Autodesk Inventor part; units mm, degrees
(part 2 of 2)
sketch "Sketch4" plane through (0, 0, 20) normal (0, 0, 1) x (1, 0, 0)
  line L0 (-68.9429, 68.9429) -> (-21.2132, 21.2132) projected
  arc A0 (-21.2132, 21.2132) -> (21.2132, -21.2132) centre (0, 0) ccw projected
  line L1 (21.2132, -21.2132) -> (68.9429, -68.9429) projected
  arc A1 (68.9429, -68.9429) -> (69.4823, -68.3993) centre (0, 0) ccw projected
  arc A2 (69.4823, -68.3993) -> (73.8041, -70.4056) centre (83.4681, -43.9299) ccw projected
  arc A3 (73.8041, -70.4056) -> (74.9009, -69.2377) centre (0, 0) ccw projected
  arc A4 (74.9009, -69.2377) -> (72.6272, -65.0503) centre (49.0843, -80.5451) ccw projected
  arc A5 (72.6272, -65.0503) -> (73.64, -63.9015) centre (0, 0) ccw projected
  arc A6 (73.64, -63.9015) -> (78.0793, -65.6325) centre (86.0618, -38.6023) ccw projected
  arc A7 (78.0793, -65.6325) -> (79.1006, -64.398) centre (0, 0) ccw projected
  arc A8 (79.1006, -64.398) -> (76.5684, -60.3617) centre (54.0449, -77.3041) ccw projected
  arc A9 (76.5684, -60.3617) -> (77.5071, -59.1515) centre (0, 0) ccw projected
  arc A10 (77.5071, -59.1515) -> (82.0463, -60.6003) centre (88.3159, -33.1222) ccw projected
  arc A11 (82.0463, -60.6003) -> (82.9881, -59.3041) centre (0, 0) ccw projected
  arc A12 (82.9881, -59.3041) -> (80.2075, -55.4348) centre (58.7922, -73.758) ccw projected
  arc A13 (80.2075, -55.4348) -> (81.0683, -54.1681) centre (0, 0) ccw projected
  arc A14 (81.0683, -54.1681) -> (85.6895, -55.329) centre (90.2213, -27.5115) ccw projected
  arc A15 (85.6895, -55.329) -> (86.548, -53.9763) centre (0, 0) ccw projected
  arc A16 (86.548, -53.9763) -> (83.53, -50.2891) centre (63.3075, -69.9209) ccw projected
  arc A17 (83.53, -50.2891) -> (84.3096, -48.9709) centre (0, 0) ccw projected
  arc A18 (84.3096, -48.9709) -> (88.9946, -49.8394) centre (91.7708, -21.7921) ccw projected
  arc A19 (88.9946, -49.8394) -> (89.7665, -48.4354) centre (0, 0) ccw projected
  arc A20 (89.7665, -48.4354) -> (86.5228, -44.945) centre (67.5729, -65.8078) ccw projected
  arc A21 (86.5228, -44.945) -> (87.2181, -43.5804) centre (0, 0) ccw projected
  arc A22 (87.2181, -43.5804) -> (91.9484, -44.153) centre (92.958, -15.9868) ccw projected
  arc A23 (91.9484, -44.153) -> (92.6306, -42.7033) centre (0, 0) ccw projected
  arc A24 (92.6306, -42.7033) -> (89.1742, -39.4235) centre (71.5717, -61.435) ccw projected
  arc A25 (89.1742, -39.4235) -> (89.7824, -38.0179) centre (0, 0) ccw projected
  arc A26 (89.7824, -38.0179) -> (94.5394, -38.2924) centre (93.7784, -10.1184) ccw projected
  arc A27 (94.5394, -38.2924) -> (95.1292, -36.8027) centre (0, 0) ccw projected
  arc A28 (95.1292, -36.8027) -> (91.4737, -33.7464) centre (75.288, -56.8198) ccw projected
  arc A29 (91.4737, -33.7464) -> (91.9924, -32.3054) centre (0, 0) ccw projected
  arc A30 (91.9924, -32.3054) -> (96.7572, -32.2807) centre (94.2287, -4.21) ccw projected
  arc A31 (96.7572, -32.2807) -> (97.2523, -30.7569) centre (0, 0) ccw projected
  arc A32 (97.2523, -30.7569) -> (93.4121, -27.9361) centre (78.7072, -51.9803) ccw projected
  arc A33 (93.4121, -27.9361) -> (93.8394, -26.4654) centre (0, 0) ccw projected
  arc A34 (93.8394, -26.4654) -> (98.5932, -26.1415) centre (94.3071, 1.715) ccw projected
  arc A35 (98.5932, -26.1415) -> (98.9917, -24.5897) centre (0, 0) ccw projected
  arc A36 (98.9917, -24.5897) -> (94.9819, -22.0156) centre (81.8157, -46.9356) ccw projected
  arc A37 (94.9819, -22.0156) -> (95.316, -20.521) centre (0, 0) ccw projected
  arc A38 (95.316, -20.521) -> (100.0401, -19.8992) centre (94.0133, 7.6332) ccw projected
  arc A39 (100.0401, -19.8992) -> (100.3403, -18.3254) centre (0, 0) ccw projected
  arc A40 (100.3403, -18.3254) -> (96.1769, -16.0082) centre (84.6014, -41.7058) ccw projected
  arc A41 (96.1769, -16.0082) -> (96.4164, -14.4956) centre (0, 0) ccw projected
  arc A42 (96.4164, -14.4956) -> (101.0922, -13.5784) centre (93.3485, 13.5213) ccw projected
  arc A43 (101.0922, -13.5784) -> (101.293, -11.9888) centre (0, 0) ccw projected
  arc A44 (101.293, -11.9888) -> (96.9922, -9.9376) centre (87.0532, -36.3113) ccw projected
  arc A45 (96.9922, -9.9376) -> (97.1364, -8.4129) centre (0, 0) ccw projected
  arc A46 (97.1364, -8.4129) -> (101.7453, -7.204) centre (92.3153, 19.356) ccw projected
  arc A47 (101.7453, -7.204) -> (101.8459, -5.6049) centre (0, 0) ccw projected
  arc A48 (101.8459, -5.6049) -> (97.4248, -3.8278) centre (89.1614, -30.7735) ccw projected
  arc A49 (97.4248, -3.8278) -> (97.4729, -2.2971) centre (0, 0) ccw projected
  arc A50 (97.4729, -2.2971) -> (101.9969, -0.8011) centre (90.9178, 25.1143) ccw projected
  arc A51 (101.9969, -0.8011) -> (101.9969, 0.8011) centre (0, 0) ccw projected
  arc A52 (101.9969, 0.8011) -> (97.4729, 2.2971) centre (90.9178, -25.1143) ccw projected
  arc A53 (97.4729, 2.2971) -> (97.4248, 3.8278) centre (0, 0) ccw projected
  arc A54 (97.4248, 3.8278) -> (101.8459, 5.6049) centre (89.1614, 30.7735) ccw projected
  arc A55 (101.8459, 5.6049) -> (101.7453, 7.204) centre (0, 0) ccw projected
  arc A56 (101.7453, 7.204) -> (97.1364, 8.4129) centre (92.3153, -19.356) ccw projected
  arc A57 (97.1364, 8.4129) -> (96.9922, 9.9376) centre (0, 0) ccw projected
  arc A58 (96.9922, 9.9376) -> (101.293, 11.9888) centre (87.0532, 36.3113) ccw projected
  arc A59 (101.293, 11.9888) -> (101.0922, 13.5784) centre (0, 0) ccw projected
  arc A60 (101.0922, 13.5784) -> (96.4164, 14.4956) centre (93.3485, -13.5213) ccw projected
  arc A61 (96.4164, 14.4956) -> (96.1769, 16.0082) centre (0, 0) ccw projected
  arc A62 (96.1769, 16.0082) -> (100.3403, 18.3254) centre (84.6014, 41.7058) ccw projected
  arc A63 (100.3403, 18.3254) -> (100.0401, 19.8992) centre (0, 0) ccw projected
  arc A64 (100.0401, 19.8992) -> (95.316, 20.521) centre (94.0133, -7.6332) ccw projected
  arc A65 (95.316, 20.521) -> (94.9819, 22.0156) centre (0, 0) ccw projected
  arc A66 (94.9819, 22.0156) -> (98.9917, 24.5897) centre (81.8157, 46.9356) ccw projected
  arc A67 (98.9917, 24.5897) -> (98.5932, 26.1415) centre (0, 0) ccw projected
  arc A68 (98.5932, 26.1415) -> (93.8394, 26.4654) centre (94.3071, -1.715) ccw projected
  arc A69 (93.8394, 26.4654) -> (93.4121, 27.9361) centre (0, 0) ccw projected
  arc A70 (93.4121, 27.9361) -> (97.2523, 30.7569) centre (78.7072, 51.9803) ccw projected
  arc A71 (97.2523, 30.7569) -> (96.7572, 32.2807) centre (0, 0) ccw projected
  arc A72 (96.7572, 32.2807) -> (91.9924, 32.3054) centre (94.2287, 4.21) ccw projected
  arc A73 (91.9924, 32.3054) -> (91.4737, 33.7464) centre (0, 0) ccw projected
  arc A74 (91.4737, 33.7464) -> (95.1292, 36.8027) centre (75.288, 56.8198) ccw projected
  arc A75 (95.1292, 36.8027) -> (94.5394, 38.2924) centre (0, 0) ccw projected
  arc A76 (94.5394, 38.2924) -> (89.7824, 38.0179) centre (93.7784, 10.1184) ccw projected
  arc A77 (89.7824, 38.0179) -> (89.1742, 39.4235) centre (0, 0) ccw projected
  arc A78 (89.1742, 39.4235) -> (92.6306, 42.7033) centre (71.5717, 61.435) ccw projected
  arc A79 (92.6306, 42.7033) -> (91.9484, 44.153) centre (0, 0) ccw projected
  arc A80 (91.9484, 44.153) -> (87.2181, 43.5804) centre (92.958, 15.9868) ccw projected
  arc A81 (87.2181, 43.5804) -> (86.5228, 44.945) centre (0, 0) ccw projected
  arc A82 (86.5228, 44.945) -> (89.7665, 48.4354) centre (67.5729, 65.8078) ccw projected
  arc A83 (89.7665, 48.4354) -> (88.9946, 49.8394) centre (0, 0) ccw projected
  arc A84 (88.9946, 49.8394) -> (84.3096, 48.9709) centre (91.7708, 21.7921) ccw projected
  arc A85 (84.3096, 48.9709) -> (83.53, 50.2891) centre (0, 0) ccw projected
  arc A86 (83.53, 50.2891) -> (86.548, 53.9763) centre (63.3075, 69.9209) ccw projected
  arc A87 (86.548, 53.9763) -> (85.6895, 55.329) centre (0, 0) ccw projected
  arc A88 (85.6895, 55.329) -> (81.0683, 54.1681) centre (90.2213, 27.5115) ccw projected
  arc A89 (81.0683, 54.1681) -> (80.2075, 55.4348) centre (0, 0) ccw projected
  arc A90 (80.2075, 55.4348) -> (82.9881, 59.3041) centre (58.7922, 73.758) ccw projected
  arc A91 (82.9881, 59.3041) -> (82.0463, 60.6003) centre (0, 0) ccw projected
  arc A92 (82.0463, 60.6003) -> (77.5071, 59.1515) centre (88.3159, 33.1222) ccw projected
  arc A93 (77.5071, 59.1515) -> (76.5684, 60.3617) centre (0, 0) ccw projected
  arc A94 (76.5684, 60.3617) -> (79.1006, 64.398) centre (54.0449, 77.3041) ccw projected
  arc A95 (79.1006, 64.398) -> (78.0793, 65.6325) centre (0, 0) ccw projected
  arc A96 (78.0793, 65.6325) -> (73.64, 63.9015) centre (86.0618, 38.6023) ccw projected
  arc A97 (73.64, 63.9015) -> (72.6272, 65.0503) centre (0, 0) ccw projected
  arc A98 (72.6272, 65.0503) -> (74.9009, 69.2377) centre (49.0843, 80.5451) ccw projected
  arc A99 (74.9009, 69.2377) -> (73.8041, 70.4056) centre (0, 0) ccw projected
  arc A100 (73.8041, 70.4056) -> (69.4823, 68.3993) centre (83.4681, 43.9299) ccw projected
  arc A101 (69.4823, 68.3993) -> (68.3993, 69.4823) centre (0, 0) ccw projected
  arc A102 (68.3993, 69.4823) -> (70.4056, 73.8041) centre (43.9299, 83.4681) ccw projected
  arc A103 (70.4056, 73.8041) -> (69.2377, 74.9009) centre (0, 0) ccw projected
  arc A104 (69.2377, 74.9009) -> (65.0503, 72.6272) centre (80.5451, 49.0843) ccw projected
  arc A105 (65.0503, 72.6272) -> (63.9015, 73.64) centre (0, 0) ccw projected
  arc A106 (63.9015, 73.64) -> (65.6325, 78.0793) centre (38.6023, 86.0618) ccw projected
  arc A107 (65.6325, 78.0793) -> (64.398, 79.1006) centre (0, 0) ccw projected
  arc A108 (64.398, 79.1006) -> (60.3617, 76.5684) centre (77.3041, 54.0449) ccw projected
  arc A109 (60.3617, 76.5684) -> (59.1515, 77.5071) centre (0, 0) ccw projected
  arc A110 (59.1515, 77.5071) -> (60.6003, 82.0463) centre (33.1222, 88.3159) ccw projected
  arc A111 (60.6003, 82.0463) -> (59.3041, 82.9881) centre (0, 0) ccw projected
  arc A112 (59.3041, 82.9881) -> (55.4348, 80.2075) centre (73.758, 58.7922) ccw projected
  arc A113 (55.4348, 80.2075) -> (54.1681, 81.0683) centre (0, 0) ccw projected
  arc A114 (54.1681, 81.0683) -> (55.329, 85.6895) centre (27.5115, 90.2213) ccw projected
  arc A115 (55.329, 85.6895) -> (53.9763, 86.548) centre (0, 0) ccw projected
  arc A116 (53.9763, 86.548) -> (50.2891, 83.53) centre (69.9209, 63.3075) ccw projected
  arc A117 (50.2891, 83.53) -> (48.9709, 84.3096) centre (0, 0) ccw projected
  arc A118 (48.9709, 84.3096) -> (49.8394, 88.9946) centre (21.7921, 91.7708) ccw projected
  arc A119 (49.8394, 88.9946) -> (48.4354, 89.7665) centre (0, 0) ccw projected
  arc A120 (48.4354, 89.7665) -> (44.945, 86.5228) centre (65.8078, 67.5729) ccw projected
  arc A121 (44.945, 86.5228) -> (43.5804, 87.2181) centre (0, 0) ccw projected
  arc A122 (43.5804, 87.2181) -> (44.153, 91.9484) centre (15.9868, 92.958) ccw projected
  arc A123 (44.153, 91.9484) -> (42.7033, 92.6306) centre (0, 0) ccw projected
  arc A124 (42.7033, 92.6306) -> (39.4235, 89.1742) centre (61.435, 71.5717) ccw projected
  arc A125 (39.4235, 89.1742) -> (38.0179, 89.7824) centre (0, 0) ccw projected
  arc A126 (38.0179, 89.7824) -> (38.2924, 94.5394) centre (10.1184, 93.7784) ccw projected
  arc A127 (38.2924, 94.5394) -> (36.8027, 95.1292) centre (0, 0) ccw projected
  arc A128 (36.8027, 95.1292) -> (33.7464, 91.4737) centre (56.8198, 75.288) ccw projected
  arc A129 (33.7464, 91.4737) -> (32.3054, 91.9924) centre (0, 0) ccw projected
  arc A130 (32.3054, 91.9924) -> (32.2807, 96.7572) centre (4.21, 94.2287) ccw projected
  arc A131 (32.2807, 96.7572) -> (30.7569, 97.2523) centre (0, 0) ccw projected
  arc A132 (30.7569, 97.2523) -> (27.9361, 93.4121) centre (51.9803, 78.7072) ccw projected
  arc A133 (27.9361, 93.4121) -> (26.4654, 93.8394) centre (0, 0) ccw projected
  arc A134 (26.4654, 93.8394) -> (26.1415, 98.5932) centre (-1.715, 94.3071) ccw projected
  arc A135 (26.1415, 98.5932) -> (24.5897, 98.9917) centre (0, 0) ccw projected
  arc A136 (24.5897, 98.9917) -> (22.0156, 94.9819) centre (46.9356, 81.8157) ccw projected
  arc A137 (22.0156, 94.9819) -> (20.521, 95.316) centre (0, 0) ccw projected
  arc A138 (20.521, 95.316) -> (19.8992, 100.0401) centre (-7.6332, 94.0133) ccw projected
  arc A139 (19.8992, 100.0401) -> (18.3254, 100.3403) centre (0, 0) ccw projected
  arc A140 (18.3254, 100.3403) -> (16.0082, 96.1769) centre (41.7058, 84.6014) ccw projected
  arc A141 (16.0082, 96.1769) -> (14.4956, 96.4164) centre (0, 0) ccw projected
  arc A142 (14.4956, 96.4164) -> (13.5784, 101.0922) centre (-13.5213, 93.3485) ccw projected
  arc A143 (13.5784, 101.0922) -> (11.9888, 101.293) centre (0, 0) ccw projected
  arc A144 (11.9888, 101.293) -> (9.9376, 96.9922) centre (36.3113, 87.0532) ccw projected
  arc A145 (9.9376, 96.9922) -> (8.4129, 97.1364) centre (0, 0) ccw projected
  arc A146 (8.4129, 97.1364) -> (7.204, 101.7453) centre (-19.356, 92.3153) ccw projected
  arc A147 (7.204, 101.7453) -> (5.6049, 101.8459) centre (0, 0) ccw projected
  arc A148 (5.6049, 101.8459) -> (3.8278, 97.4248) centre (30.7735, 89.1614) ccw projected
  arc A149 (3.8278, 97.4248) -> (2.2971, 97.4729) centre (0, 0) ccw projected
  arc A150 (2.2971, 97.4729) -> (0.8011, 101.9969) centre (-25.1143, 90.9178) ccw projected
  arc A151 (0.8011, 101.9969) -> (-0.8011, 101.9969) centre (0, 0) ccw projected
  arc A152 (-0.8011, 101.9969) -> (-2.2971, 97.4729) centre (25.1143, 90.9178) ccw projected
  arc A153 (-2.2971, 97.4729) -> (-3.8278, 97.4248) centre (0, 0) ccw projected
  arc A154 (-3.8278, 97.4248) -> (-5.6049, 101.8459) centre (-30.7735, 89.1614) ccw projected
  arc A155 (-5.6049, 101.8459) -> (-7.204, 101.7453) centre (0, 0) ccw projected
  arc A156 (-7.204, 101.7453) -> (-8.4129, 97.1364) centre (19.356, 92.3153) ccw projected
  arc A157 (-8.4129, 97.1364) -> (-9.9376, 96.9922) centre (0, 0) ccw projected
  arc A158 (-9.9376, 96.9922) -> (-11.9888, 101.293) centre (-36.3113, 87.0532) ccw projected
  arc A159 (-11.9888, 101.293) -> (-13.5784, 101.0922) centre (0, 0) ccw projected
  arc A160 (-13.5784, 101.0922) -> (-14.4956, 96.4164) centre (13.5213, 93.3485) ccw projected
  arc A161 (-14.4956, 96.4164) -> (-16.0082, 96.1769) centre (0, 0) ccw projected
  arc A162 (-16.0082, 96.1769) -> (-18.3254, 100.3403) centre (-41.7058, 84.6014) ccw projected
  arc A163 (-18.3254, 100.3403) -> (-19.8992, 100.0401) centre (0, 0) ccw projected
  arc A164 (-19.8992, 100.0401) -> (-20.521, 95.316) centre (7.6332, 94.0133) ccw projected
  arc A165 (-20.521, 95.316) -> (-22.0156, 94.9819) centre (0, 0) ccw projected
  arc A166 (-22.0156, 94.9819) -> (-24.5897, 98.9917) centre (-46.9356, 81.8157) ccw projected
  arc A167 (-24.5897, 98.9917) -> (-26.1415, 98.5932) centre (0, 0) ccw projected
  arc A168 (-26.1415, 98.5932) -> (-26.4654, 93.8394) centre (1.715, 94.3071) ccw projected
  arc A169 (-26.4654, 93.8394) -> (-27.9361, 93.4121) centre (0, 0) ccw projected
  arc A170 (-27.9361, 93.4121) -> (-30.7569, 97.2523) centre (-51.9803, 78.7072) ccw projected
  arc A171 (-30.7569, 97.2523) -> (-32.2807, 96.7572) centre (0, 0) ccw projected
  arc A172 (-32.2807, 96.7572) -> (-32.3054, 91.9924) centre (-4.21, 94.2287) ccw projected
  arc A173 (-32.3054, 91.9924) -> (-33.7464, 91.4737) centre (0, 0) ccw projected
  arc A174 (-33.7464, 91.4737) -> (-36.8027, 95.1292) centre (-56.8198, 75.288) ccw projected
  arc A175 (-36.8027, 95.1292) -> (-38.2924, 94.5394) centre (0, 0) ccw projected
  arc A176 (-38.2924, 94.5394) -> (-38.0179, 89.7824) centre (-10.1184, 93.7784) ccw projected
  arc A177 (-38.0179, 89.7824) -> (-39.4235, 89.1742) centre (0, 0) ccw projected
  arc A178 (-39.4235, 89.1742) -> (-42.7033, 92.6306) centre (-61.435, 71.5717) ccw projected
  arc A179 (-42.7033, 92.6306) -> (-44.153, 91.9484) centre (0, 0) ccw projected
  arc A180 (-44.153, 91.9484) -> (-43.5804, 87.2181) centre (-15.9868, 92.958) ccw projected
  arc A181 (-43.5804, 87.2181) -> (-44.945, 86.5228) centre (0, 0) ccw projected
  arc A182 (-44.945, 86.5228) -> (-48.4354, 89.7665) centre (-65.8078, 67.5729) ccw projected
  arc A183 (-48.4354, 89.7665) -> (-49.8394, 88.9946) centre (0, 0) ccw projected
  arc A184 (-49.8394, 88.9946) -> (-48.9709, 84.3096) centre (-21.7921, 91.7708) ccw projected
  arc A185 (-48.9709, 84.3096) -> (-50.2891, 83.53) centre (0, 0) ccw projected
  arc A186 (-50.2891, 83.53) -> (-53.9763, 86.548) centre (-69.9209, 63.3075) ccw projected
  arc A187 (-53.9763, 86.548) -> (-55.329, 85.6895) centre (0, 0) ccw projected
  arc A188 (-55.329, 85.6895) -> (-54.1681, 81.0683) centre (-27.5115, 90.2213) ccw projected
  arc A189 (-54.1681, 81.0683) -> (-55.4348, 80.2075) centre (0, 0) ccw projected
  arc A190 (-55.4348, 80.2075) -> (-59.3041, 82.9881) centre (-73.758, 58.7922) ccw projected
  arc A191 (-59.3041, 82.9881) -> (-60.6003, 82.0463) centre (0, 0) ccw projected
  arc A192 (-60.6003, 82.0463) -> (-59.1515, 77.5071) centre (-33.1222, 88.3159) ccw projected
  arc A193 (-59.1515, 77.5071) -> (-60.3617, 76.5684) centre (0, 0) ccw projected
  arc A194 (-60.3617, 76.5684) -> (-64.398, 79.1006) centre (-77.3041, 54.0449) ccw projected
  arc A195 (-64.398, 79.1006) -> (-65.6325, 78.0793) centre (0, 0) ccw projected
  arc A196 (-65.6325, 78.0793) -> (-63.9015, 73.64) centre (-38.6023, 86.0618) ccw projected
  arc A197 (-63.9015, 73.64) -> (-65.0503, 72.6272) centre (0, 0) ccw projected
  arc A198 (-65.0503, 72.6272) -> (-69.2377, 74.9009) centre (-80.5451, 49.0843) ccw projected
  arc A199 (-69.2377, 74.9009) -> (-70.4056, 73.8041) centre (0, 0) ccw projected
  arc A200 (-70.4056, 73.8041) -> (-68.3993, 69.4823) centre (-43.9299, 83.4681) ccw projected
  arc A201 (-68.3993, 69.4823) -> (-68.9429, 68.9429) centre (0, 0) ccw projected
  circle A202 centre (0, 0) radius 10 projected
  line L2 (0, 0) -> (21.2132, 21.2132)
  line L3 (0, 0) -> (30, 0) construction
  circle A203 centre (21.2132, 21.2132) radius 10
  dimension "d55" = 30
  dimension "d56" = 45
  dimension "d57" = 20
  constraints: 4 end point, 1 centre point, 1 coincident, 1 equal length, 1 horizontal
  measures "d55" distance of L2.start L2.end
  measures "d56" angle of L3 L2
  measures "d57" diameter of A203
extrude "Extrusion3" cut sketch "Sketch4" against normal up to surface (20 mm away) contours A203
sketch "Sketch6" plane through (0, 0, 20) normal (0, 0, 1) x (1, 0, 0)
  circle A0 centre (21.2132, 21.2132) radius 10 projected
  line L0 (-68.9429, 68.9429) -> (-21.2132, 21.2132) projected
  arc A1 (-21.2132, 21.2132) -> (21.2132, -21.2132) centre (0, 0) ccw projected
  line L1 (21.2132, -21.2132) -> (68.9429, -68.9429) projected
  arc A2 (68.9429, -68.9429) -> (69.4823, -68.3993) centre (0, 0) ccw projected
  arc A3 (69.4823, -68.3993) -> (73.8041, -70.4056) centre (83.4681, -43.9299) ccw projected
  arc A4 (73.8041, -70.4056) -> (74.9009, -69.2377) centre (0, 0) ccw projected
  arc A5 (74.9009, -69.2377) -> (72.6272, -65.0503) centre (49.0843, -80.5451) ccw projected
  arc A6 (72.6272, -65.0503) -> (73.64, -63.9015) centre (0, 0) ccw projected
  arc A7 (73.64, -63.9015) -> (78.0793, -65.6325) centre (86.0618, -38.6023) ccw projected
  arc A8 (78.0793, -65.6325) -> (79.1006, -64.398) centre (0, 0) ccw projected
  arc A9 (79.1006, -64.398) -> (76.5684, -60.3617) centre (54.0449, -77.3041) ccw projected
  arc A10 (76.5684, -60.3617) -> (77.5071, -59.1515) centre (0, 0) ccw projected
  arc A11 (77.5071, -59.1515) -> (82.0463, -60.6003) centre (88.3159, -33.1222) ccw projected
  arc A12 (82.0463, -60.6003) -> (82.9881, -59.3041) centre (0, 0) ccw projected
  arc A13 (82.9881, -59.3041) -> (80.2075, -55.4348) centre (58.7922, -73.758) ccw projected
  arc A14 (80.2075, -55.4348) -> (81.0683, -54.1681) centre (0, 0) ccw projected
  arc A15 (81.0683, -54.1681) -> (85.6895, -55.329) centre (90.2213, -27.5115) ccw projected
  arc A16 (85.6895, -55.329) -> (86.548, -53.9763) centre (0, 0) ccw projected
  arc A17 (86.548, -53.9763) -> (83.53, -50.2891) centre (63.3075, -69.9209) ccw projected
  arc A18 (83.53, -50.2891) -> (84.3096, -48.9709) centre (0, 0) ccw projected
  arc A19 (84.3096, -48.9709) -> (88.9946, -49.8394) centre (91.7708, -21.7921) ccw projected
  arc A20 (88.9946, -49.8394) -> (89.7665, -48.4354) centre (0, 0) ccw projected
  arc A21 (89.7665, -48.4354) -> (86.5228, -44.945) centre (67.5729, -65.8078) ccw projected
  arc A22 (86.5228, -44.945) -> (87.2181, -43.5804) centre (0, 0) ccw projected
  arc A23 (87.2181, -43.5804) -> (91.9484, -44.153) centre (92.958, -15.9868) ccw projected
  arc A24 (91.9484, -44.153) -> (92.6306, -42.7033) centre (0, 0) ccw projected
  arc A25 (92.6306, -42.7033) -> (89.1742, -39.4235) centre (71.5717, -61.435) ccw projected
  arc A26 (89.1742, -39.4235) -> (89.7824, -38.0179) centre (0, 0) ccw projected
  arc A27 (89.7824, -38.0179) -> (94.5394, -38.2924) centre (93.7784, -10.1184) ccw projected
  arc A28 (94.5394, -38.2924) -> (95.1292, -36.8027) centre (0, 0) ccw projected
  arc A29 (95.1292, -36.8027) -> (91.4737, -33.7464) centre (75.288, -56.8198) ccw projected
  arc A30 (91.4737, -33.7464) -> (91.9924, -32.3054) centre (0, 0) ccw projected
  arc A31 (91.9924, -32.3054) -> (96.7572, -32.2807) centre (94.2287, -4.21) ccw projected
  arc A32 (96.7572, -32.2807) -> (97.2523, -30.7569) centre (0, 0) ccw projected
  arc A33 (97.2523, -30.7569) -> (93.4121, -27.9361) centre (78.7072, -51.9803) ccw projected
  arc A34 (93.4121, -27.9361) -> (93.8394, -26.4654) centre (0, 0) ccw projected
  arc A35 (93.8394, -26.4654) -> (98.5932, -26.1415) centre (94.3071, 1.715) ccw projected
  arc A36 (98.5932, -26.1415) -> (98.9917, -24.5897) centre (0, 0) ccw projected
  arc A37 (98.9917, -24.5897) -> (94.9819, -22.0156) centre (81.8157, -46.9356) ccw projected
  arc A38 (94.9819, -22.0156) -> (95.316, -20.521) centre (0, 0) ccw projected
  arc A39 (95.316, -20.521) -> (100.0401, -19.8992) centre (94.0133, 7.6332) ccw projected
  arc A40 (100.0401, -19.8992) -> (100.3403, -18.3254) centre (0, 0) ccw projected
  arc A41 (100.3403, -18.3254) -> (96.1769, -16.0082) centre (84.6014, -41.7058) ccw projected
  arc A42 (96.1769, -16.0082) -> (96.4164, -14.4956) centre (0, 0) ccw projected
  arc A43 (96.4164, -14.4956) -> (101.0922, -13.5784) centre (93.3485, 13.5213) ccw projected
  arc A44 (101.0922, -13.5784) -> (101.293, -11.9888) centre (0, 0) ccw projected
  arc A45 (101.293, -11.9888) -> (96.9922, -9.9376) centre (87.0532, -36.3113) ccw projected
  arc A46 (96.9922, -9.9376) -> (97.1364, -8.4129) centre (0, 0) ccw projected
  arc A47 (97.1364, -8.4129) -> (101.7453, -7.204) centre (92.3153, 19.356) ccw projected
  arc A48 (101.7453, -7.204) -> (101.8459, -5.6049) centre (0, 0) ccw projected
  arc A49 (101.8459, -5.6049) -> (97.4248, -3.8278) centre (89.1614, -30.7735) ccw projected
  arc A50 (97.4248, -3.8278) -> (97.4729, -2.2971) centre (0, 0) ccw projected
  arc A51 (97.4729, -2.2971) -> (101.9969, -0.8011) centre (90.9178, 25.1143) ccw projected
  arc A52 (101.9969, -0.8011) -> (101.9969, 0.8011) centre (0, 0) ccw projected
  arc A53 (101.9969, 0.8011) -> (97.4729, 2.2971) centre (90.9178, -25.1143) ccw projected
  arc A54 (97.4729, 2.2971) -> (97.4248, 3.8278) centre (0, 0) ccw projected
  arc A55 (97.4248, 3.8278) -> (101.8459, 5.6049) centre (89.1614, 30.7735) ccw projected
  arc A56 (101.8459, 5.6049) -> (101.7453, 7.204) centre (0, 0) ccw projected
  arc A57 (101.7453, 7.204) -> (97.1364, 8.4129) centre (92.3153, -19.356) ccw projected
  arc A58 (97.1364, 8.4129) -> (96.9922, 9.9376) centre (0, 0) ccw projected
  arc A59 (96.9922, 9.9376) -> (101.293, 11.9888) centre (87.0532, 36.3113) ccw projected
  arc A60 (101.293, 11.9888) -> (101.0922, 13.5784) centre (0, 0) ccw projected
  arc A61 (101.0922, 13.5784) -> (96.4164, 14.4956) centre (93.3485, -13.5213) ccw projected
  arc A62 (96.4164, 14.4956) -> (96.1769, 16.0082) centre (0, 0) ccw projected
  arc A63 (96.1769, 16.0082) -> (100.3403, 18.3254) centre (84.6014, 41.7058) ccw projected
  arc A64 (100.3403, 18.3254) -> (100.0401, 19.8992) centre (0, 0) ccw projected
  arc A65 (100.0401, 19.8992) -> (95.316, 20.521) centre (94.0133, -7.6332) ccw projected
  arc A66 (95.316, 20.521) -> (94.9819, 22.0156) centre (0, 0) ccw projected
  arc A67 (94.9819, 22.0156) -> (98.9917, 24.5897) centre (81.8157, 46.9356) ccw projected
  arc A68 (98.9917, 24.5897) -> (98.5932, 26.1415) centre (0, 0) ccw projected
  arc A69 (98.5932, 26.1415) -> (93.8394, 26.4654) centre (94.3071, -1.715) ccw projected
  arc A70 (93.8394, 26.4654) -> (93.4121, 27.9361) centre (0, 0) ccw projected
  arc A71 (93.4121, 27.9361) -> (97.2523, 30.7569) centre (78.7072, 51.9803) ccw projected
  arc A72 (97.2523, 30.7569) -> (96.7572, 32.2807) centre (0, 0) ccw projected
  arc A73 (96.7572, 32.2807) -> (91.9924, 32.3054) centre (94.2287, 4.21) ccw projected
  arc A74 (91.9924, 32.3054) -> (91.4737, 33.7464) centre (0, 0) ccw projected
  arc A75 (91.4737, 33.7464) -> (95.1292, 36.8027) centre (75.288, 56.8198) ccw projected
  arc A76 (95.1292, 36.8027) -> (94.5394, 38.2924) centre (0, 0) ccw projected
  arc A77 (94.5394, 38.2924) -> (89.7824, 38.0179) centre (93.7784, 10.1184) ccw projected
  arc A78 (89.7824, 38.0179) -> (89.1742, 39.4235) centre (0, 0) ccw projected
  arc A79 (89.1742, 39.4235) -> (92.6306, 42.7033) centre (71.5717, 61.435) ccw projected
  arc A80 (92.6306, 42.7033) -> (91.9484, 44.153) centre (0, 0) ccw projected
  arc A81 (91.9484, 44.153) -> (87.2181, 43.5804) centre (92.958, 15.9868) ccw projected
  arc A82 (87.2181, 43.5804) -> (86.5228, 44.945) centre (0, 0) ccw projected
  arc A83 (86.5228, 44.945) -> (89.7665, 48.4354) centre (67.5729, 65.8078) ccw projected
  arc A84 (89.7665, 48.4354) -> (88.9946, 49.8394) centre (0, 0) ccw projected
  arc A85 (88.9946, 49.8394) -> (84.3096, 48.9709) centre (91.7708, 21.7921) ccw projected
  arc A86 (84.3096, 48.9709) -> (83.53, 50.2891) centre (0, 0) ccw projected
  arc A87 (83.53, 50.2891) -> (86.548, 53.9763) centre (63.3075, 69.9209) ccw projected
  arc A88 (86.548, 53.9763) -> (85.6895, 55.329) centre (0, 0) ccw projected
  arc A89 (85.6895, 55.329) -> (81.0683, 54.1681) centre (90.2213, 27.5115) ccw projected
  arc A90 (81.0683, 54.1681) -> (80.2075, 55.4348) centre (0, 0) ccw projected
  arc A91 (80.2075, 55.4348) -> (82.9881, 59.3041) centre (58.7922, 73.758) ccw projected
  arc A92 (82.9881, 59.3041) -> (82.0463, 60.6003) centre (0, 0) ccw projected
  arc A93 (82.0463, 60.6003) -> (77.5071, 59.1515) centre (88.3159, 33.1222) ccw projected
  arc A94 (77.5071, 59.1515) -> (76.5684, 60.3617) centre (0, 0) ccw projected
  arc A95 (76.5684, 60.3617) -> (79.1006, 64.398) centre (54.0449, 77.3041) ccw projected
  arc A96 (79.1006, 64.398) -> (78.0793, 65.6325) centre (0, 0) ccw projected
  arc A97 (78.0793, 65.6325) -> (73.64, 63.9015) centre (86.0618, 38.6023) ccw projected
  arc A98 (73.64, 63.9015) -> (72.6272, 65.0503) centre (0, 0) ccw projected
  arc A99 (72.6272, 65.0503) -> (74.9009, 69.2377) centre (49.0843, 80.5451) ccw projected
  arc A100 (74.9009, 69.2377) -> (73.8041, 70.4056) centre (0, 0) ccw projected
  arc A101 (73.8041, 70.4056) -> (69.4823, 68.3993) centre (83.4681, 43.9299) ccw projected
  arc A102 (69.4823, 68.3993) -> (68.3993, 69.4823) centre (0, 0) ccw projected
  arc A103 (68.3993, 69.4823) -> (70.4056, 73.8041) centre (43.9299, 83.4681) ccw projected
  arc A104 (70.4056, 73.8041) -> (69.2377, 74.9009) centre (0, 0) ccw projected
  arc A105 (69.2377, 74.9009) -> (65.0503, 72.6272) centre (80.5451, 49.0843) ccw projected
  arc A106 (65.0503, 72.6272) -> (63.9015, 73.64) centre (0, 0) ccw projected
  arc A107 (63.9015, 73.64) -> (65.6325, 78.0793) centre (38.6023, 86.0618) ccw projected
  arc A108 (65.6325, 78.0793) -> (64.398, 79.1006) centre (0, 0) ccw projected
  arc A109 (64.398, 79.1006) -> (60.3617, 76.5684) centre (77.3041, 54.0449) ccw projected
  arc A110 (60.3617, 76.5684) -> (59.1515, 77.5071) centre (0, 0) ccw projected
  arc A111 (59.1515, 77.5071) -> (60.6003, 82.0463) centre (33.1222, 88.3159) ccw projected
  arc A112 (60.6003, 82.0463) -> (59.3041, 82.9881) centre (0, 0) ccw projected
  arc A113 (59.3041, 82.9881) -> (55.4348, 80.2075) centre (73.758, 58.7922) ccw projected
  arc A114 (55.4348, 80.2075) -> (54.1681, 81.0683) centre (0, 0) ccw projected
  arc A115 (54.1681, 81.0683) -> (55.329, 85.6895) centre (27.5115, 90.2213) ccw projected
  arc A116 (55.329, 85.6895) -> (53.9763, 86.548) centre (0, 0) ccw projected
  arc A117 (53.9763, 86.548) -> (50.2891, 83.53) centre (69.9209, 63.3075) ccw projected
  arc A118 (50.2891, 83.53) -> (48.9709, 84.3096) centre (0, 0) ccw projected
  arc A119 (48.9709, 84.3096) -> (49.8394, 88.9946) centre (21.7921, 91.7708) ccw projected
  arc A120 (49.8394, 88.9946) -> (48.4354, 89.7665) centre (0, 0) ccw projected
  arc A121 (48.4354, 89.7665) -> (44.945, 86.5228) centre (65.8078, 67.5729) ccw projected
  arc A122 (44.945, 86.5228) -> (43.5804, 87.2181) centre (0, 0) ccw projected
  arc A123 (43.5804, 87.2181) -> (44.153, 91.9484) centre (15.9868, 92.958) ccw projected
  arc A124 (44.153, 91.9484) -> (42.7033, 92.6306) centre (0, 0) ccw projected
  arc A125 (42.7033, 92.6306) -> (39.4235, 89.1742) centre (61.435, 71.5717) ccw projected
  arc A126 (39.4235, 89.1742) -> (38.0179, 89.7824) centre (0, 0) ccw projected
  arc A127 (38.0179, 89.7824) -> (38.2924, 94.5394) centre (10.1184, 93.7784) ccw projected
  arc A128 (38.2924, 94.5394) -> (36.8027, 95.1292) centre (0, 0) ccw projected
  arc A129 (36.8027, 95.1292) -> (33.7464, 91.4737) centre (56.8198, 75.288) ccw projected
  arc A130 (33.7464, 91.4737) -> (32.3054, 91.9924) centre (0, 0) ccw projected
  arc A131 (32.3054, 91.9924) -> (32.2807, 96.7572) centre (4.21, 94.2287) ccw projected
  arc A132 (32.2807, 96.7572) -> (30.7569, 97.2523) centre (0, 0) ccw projected
  arc A133 (30.7569, 97.2523) -> (27.9361, 93.4121) centre (51.9803, 78.7072) ccw projected
  arc A134 (27.9361, 93.4121) -> (26.4654, 93.8394) centre (0, 0) ccw projected
  arc A135 (26.4654, 93.8394) -> (26.1415, 98.5932) centre (-1.715, 94.3071) ccw projected
  arc A136 (26.1415, 98.5932) -> (24.5897, 98.9917) centre (0, 0) ccw projected
  arc A137 (24.5897, 98.9917) -> (22.0156, 94.9819) centre (46.9356, 81.8157) ccw projected
  arc A138 (22.0156, 94.9819) -> (20.521, 95.316) centre (0, 0) ccw projected
  arc A139 (20.521, 95.316) -> (19.8992, 100.0401) centre (-7.6332, 94.0133) ccw projected
  arc A140 (19.8992, 100.0401) -> (18.3254, 100.3403) centre (0, 0) ccw projected
  arc A141 (18.3254, 100.3403) -> (16.0082, 96.1769) centre (41.7058, 84.6014) ccw projected
  arc A142 (16.0082, 96.1769) -> (14.4956, 96.4164) centre (0, 0) ccw projected
  arc A143 (14.4956, 96.4164) -> (13.5784, 101.0922) centre (-13.5213, 93.3485) ccw projected
  arc A144 (13.5784, 101.0922) -> (11.9888, 101.293) centre (0, 0) ccw projected
  arc A145 (11.9888, 101.293) -> (9.9376, 96.9922) centre (36.3113, 87.0532) ccw projected
  arc A146 (9.9376, 96.9922) -> (8.4129, 97.1364) centre (0, 0) ccw projected
  arc A147 (8.4129, 97.1364) -> (7.204, 101.7453) centre (-19.356, 92.3153) ccw projected
  arc A148 (7.204, 101.7453) -> (5.6049, 101.8459) centre (0, 0) ccw projected
  arc A149 (5.6049, 101.8459) -> (3.8278, 97.4248) centre (30.7735, 89.1614) ccw projected
  arc A150 (3.8278, 97.4248) -> (2.2971, 97.4729) centre (0, 0) ccw projected
  arc A151 (2.2971, 97.4729) -> (0.8011, 101.9969) centre (-25.1143, 90.9178) ccw projected
  arc A152 (0.8011, 101.9969) -> (-0.8011, 101.9969) centre (0, 0) ccw projected
  arc A153 (-0.8011, 101.9969) -> (-2.2971, 97.4729) centre (25.1143, 90.9178) ccw projected
  arc A154 (-2.2971, 97.4729) -> (-3.8278, 97.4248) centre (0, 0) ccw projected
  arc A155 (-3.8278, 97.4248) -> (-5.6049, 101.8459) centre (-30.7735, 89.1614) ccw projected
  arc A156 (-5.6049, 101.8459) -> (-7.204, 101.7453) centre (0, 0) ccw projected
  arc A157 (-7.204, 101.7453) -> (-8.4129, 97.1364) centre (19.356, 92.3153) ccw projected
  arc A158 (-8.4129, 97.1364) -> (-9.9376, 96.9922) centre (0, 0) ccw projected
  arc A159 (-9.9376, 96.9922) -> (-11.9888, 101.293) centre (-36.3113, 87.0532) ccw projected
  arc A160 (-11.9888, 101.293) -> (-13.5784, 101.0922) centre (0, 0) ccw projected
  arc A161 (-13.5784, 101.0922) -> (-14.4956, 96.4164) centre (13.5213, 93.3485) ccw projected
  arc A162 (-14.4956, 96.4164) -> (-16.0082, 96.1769) centre (0, 0) ccw projected
  arc A163 (-16.0082, 96.1769) -> (-18.3254, 100.3403) centre (-41.7058, 84.6014) ccw projected
  arc A164 (-18.3254, 100.3403) -> (-19.8992, 100.0401) centre (0, 0) ccw projected
  arc A165 (-19.8992, 100.0401) -> (-20.521, 95.316) centre (7.6332, 94.0133) ccw projected
  arc A166 (-20.521, 95.316) -> (-22.0156, 94.9819) centre (0, 0) ccw projected
  arc A167 (-22.0156, 94.9819) -> (-24.5897, 98.9917) centre (-46.9356, 81.8157) ccw projected
  arc A168 (-24.5897, 98.9917) -> (-26.1415, 98.5932) centre (0, 0) ccw projected
  arc A169 (-26.1415, 98.5932) -> (-26.4654, 93.8394) centre (1.715, 94.3071) ccw projected
  arc A170 (-26.4654, 93.8394) -> (-27.9361, 93.4121) centre (0, 0) ccw projected
  arc A171 (-27.9361, 93.4121) -> (-30.7569, 97.2523) centre (-51.9803, 78.7072) ccw projected
  arc A172 (-30.7569, 97.2523) -> (-32.2807, 96.7572) centre (0, 0) ccw projected
  arc A173 (-32.2807, 96.7572) -> (-32.3054, 91.9924) centre (-4.21, 94.2287) ccw projected
  arc A174 (-32.3054, 91.9924) -> (-33.7464, 91.4737) centre (0, 0) ccw projected
  arc A175 (-33.7464, 91.4737) -> (-36.8027, 95.1292) centre (-56.8198, 75.288) ccw projected
  arc A176 (-36.8027, 95.1292) -> (-38.2924, 94.5394) centre (0, 0) ccw projected
  arc A177 (-38.2924, 94.5394) -> (-38.0179, 89.7824) centre (-10.1184, 93.7784) ccw projected
  arc A178 (-38.0179, 89.7824) -> (-39.4235, 89.1742) centre (0, 0) ccw projected
  arc A179 (-39.4235, 89.1742) -> (-42.7033, 92.6306) centre (-61.435, 71.5717) ccw projected
  arc A180 (-42.7033, 92.6306) -> (-44.153, 91.9484) centre (0, 0) ccw projected
  arc A181 (-44.153, 91.9484) -> (-43.5804, 87.2181) centre (-15.9868, 92.958) ccw projected
  arc A182 (-43.5804, 87.2181) -> (-44.945, 86.5228) centre (0, 0) ccw projected
  arc A183 (-44.945, 86.5228) -> (-48.4354, 89.7665) centre (-65.8078, 67.5729) ccw projected
  arc A184 (-48.4354, 89.7665) -> (-49.8394, 88.9946) centre (0, 0) ccw projected
  arc A185 (-49.8394, 88.9946) -> (-48.9709, 84.3096) centre (-21.7921, 91.7708) ccw projected
  arc A186 (-48.9709, 84.3096) -> (-50.2891, 83.53) centre (0, 0) ccw projected
  arc A187 (-50.2891, 83.53) -> (-53.9763, 86.548) centre (-69.9209, 63.3075) ccw projected
  arc A188 (-53.9763, 86.548) -> (-55.329, 85.6895) centre (0, 0) ccw projected
  arc A189 (-55.329, 85.6895) -> (-54.1681, 81.0683) centre (-27.5115, 90.2213) ccw projected
  arc A190 (-54.1681, 81.0683) -> (-55.4348, 80.2075) centre (0, 0) ccw projected
  arc A191 (-55.4348, 80.2075) -> (-59.3041, 82.9881) centre (-73.758, 58.7922) ccw projected
  arc A192 (-59.3041, 82.9881) -> (-60.6003, 82.0463) centre (0, 0) ccw projected
  arc A193 (-60.6003, 82.0463) -> (-59.1515, 77.5071) centre (-33.1222, 88.3159) ccw projected
  arc A194 (-59.1515, 77.5071) -> (-60.3617, 76.5684) centre (0, 0) ccw projected
  arc A195 (-60.3617, 76.5684) -> (-64.398, 79.1006) centre (-77.3041, 54.0449) ccw projected
  arc A196 (-64.398, 79.1006) -> (-65.6325, 78.0793) centre (0, 0) ccw projected
  arc A197 (-65.6325, 78.0793) -> (-63.9015, 73.64) centre (-38.6023, 86.0618) ccw projected
  arc A198 (-63.9015, 73.64) -> (-65.0503, 72.6272) centre (0, 0) ccw projected
  arc A199 (-65.0503, 72.6272) -> (-69.2377, 74.9009) centre (-80.5451, 49.0843) ccw projected
  arc A200 (-69.2377, 74.9009) -> (-70.4056, 73.8041) centre (0, 0) ccw projected
  arc A201 (-70.4056, 73.8041) -> (-68.3993, 69.4823) centre (-43.9299, 83.4681) ccw projected
  arc A202 (-68.3993, 69.4823) -> (-68.9429, 68.9429) centre (0, 0) ccw projected
  circle A203 centre (0, 0) radius 10 projected
  circle A204 centre (0, 0) radius 85
  line L2 (-68.9429, 68.9429) -> (-21.2132, 21.2132) projected
  circle A205 centre (-60.1041, 60.1041) radius 2
  circle A206 centre (-57.9455, 62.1878) radius 2
  circle A207 centre (-55.7147, 64.194) radius 2
  circle A208 centre (-53.4145, 66.1203) radius 2
  circle A209 centre (-51.0477, 67.9642) radius 2
  circle A210 centre (-48.6174, 69.7234) radius 2
  circle A211 centre (-46.1264, 71.3957) radius 2
  circle A212 centre (-43.578, 72.9791) radius 2
  circle A213 centre (-40.9754, 74.4716) radius 2
  circle A214 centre (-38.3216, 75.8713) radius 2
  circle A215 centre (-35.6201, 77.1765) radius 2
  circle A216 centre (-32.8743, 78.3855) radius 2
  circle A217 centre (-30.0875, 79.4968) radius 2
  circle A218 centre (-27.2632, 80.5091) radius 2
  circle A219 centre (-24.4049, 81.4211) radius 2
  circle A220 centre (-21.5162, 82.2317) radius 2
  circle A221 centre (-18.6007, 82.9398) radius 2
  circle A222 centre (-15.6621, 83.5446) radius 2
  circle A223 centre (-12.7039, 84.0453) radius 2
  circle A224 centre (-9.7299, 84.4413) radius 2
  circle A225 centre (-6.7438, 84.7321) radius 2
  circle A226 centre (-3.7493, 84.9173) radius 2
  circle A227 centre (-0.7501, 84.9967) radius 2
  circle A228 centre (2.25, 84.9702) radius 2
  circle A229 centre (5.2474, 84.8379) radius 2
  circle A230 centre (8.2381, 84.5998) radius 2
  circle A231 centre (11.2187, 84.2564) radius 2
  circle A232 centre (14.1852, 83.808) radius 2
  circle A233 centre (17.1341, 83.2552) radius 2
  circle A234 centre (20.0616, 82.5986) radius 2
  circle A235 centre (22.9641, 81.8392) radius 2
  circle A236 centre (25.838, 80.9777) radius 2
  circle A237 centre (28.6798, 80.0154) radius 2
  circle A238 centre (31.4858, 78.9534) radius 2
  circle A239 centre (34.2525, 77.7931) radius 2
  circle A240 centre (36.9766, 76.5358) radius 2
  circle A241 centre (39.6547, 75.1832) radius 2
  circle A242 centre (42.2833, 73.7369) radius 2
  circle A243 centre (44.8592, 72.1987) radius 2
  circle A244 centre (47.3793, 70.5706) radius 2
  circle A245 centre (49.8403, 68.8545) radius 2
  circle A246 centre (52.2392, 67.0527) radius 2
  circle A247 centre (54.5731, 65.1673) radius 2
  circle A248 centre (56.8389, 63.2008) radius 2
  circle A249 centre (59.034, 61.1555) radius 2
  circle A250 centre (61.1555, 59.034) radius 2
  circle A251 centre (63.2008, 56.8389) radius 2
  circle A252 centre (65.1673, 54.5731) radius 2
  circle A253 centre (67.0527, 52.2392) radius 2
  circle A254 centre (68.8545, 49.8403) radius 2
  circle A255 centre (70.5706, 47.3793) radius 2
  circle A256 centre (72.1987, 44.8592) radius 2
  circle A257 centre (73.7369, 42.2833) radius 2
  circle A258 centre (75.1832, 39.6547) radius 2
  circle A259 centre (76.5358, 36.9766) radius 2
  circle A260 centre (77.7931, 34.2525) radius 2
  circle A261 centre (78.9534, 31.4858) radius 2
  circle A262 centre (80.0154, 28.6798) radius 2
  circle A263 centre (80.9777, 25.838) radius 2
  circle A264 centre (81.8392, 22.9641) radius 2
  circle A265 centre (82.5986, 20.0616) radius 2
  circle A266 centre (83.2552, 17.1341) radius 2
  circle A267 centre (83.808, 14.1852) radius 2
  circle A268 centre (84.2564, 11.2187) radius 2
  circle A269 centre (84.5998, 8.2381) radius 2
  circle A270 centre (84.8379, 5.2474) radius 2
  circle A271 centre (84.9702, 2.25) radius 2
  circle A272 centre (84.9967, -0.7501) radius 2
  circle A273 centre (84.9173, -3.7493) radius 2
  circle A274 centre (84.7321, -6.7438) radius 2
  circle A275 centre (84.4413, -9.7299) radius 2
  circle A276 centre (84.0453, -12.7039) radius 2
  circle A277 centre (83.5446, -15.6621) radius 2
  circle A278 centre (82.9398, -18.6007) radius 2
  circle A279 centre (82.2317, -21.5162) radius 2
  circle A280 centre (81.4211, -24.4049) radius 2
  circle A281 centre (80.5091, -27.2632) radius 2
  circle A282 centre (79.4968, -30.0875) radius 2
  circle A283 centre (78.3855, -32.8743) radius 2
  circle A284 centre (77.1765, -35.6201) radius 2
  circle A285 centre (75.8713, -38.3216) radius 2
  circle A286 centre (74.4716, -40.9754) radius 2
  circle A287 centre (72.9791, -43.578) radius 2
  circle A288 centre (71.3957, -46.1264) radius 2
  circle A289 centre (69.7234, -48.6174) radius 2
  circle A290 centre (67.9642, -51.0477) radius 2
  circle A291 centre (66.1203, -53.4145) radius 2
  circle A292 centre (64.194, -55.7147) radius 2
  circle A293 centre (62.1878, -57.9455) radius 2
  circle A294 centre (60.1041, -60.1041) radius 2
  point P0 (76.9657, 36.0734)
  point P1 (78.5774, 32.4128)
  point P2 (80.3474, 27.7361)
  point P3 (81.5632, 23.9257)
  dimension "d60" = 170
  dimension "d61" = 4
  dimension "d68" = 180
  constraints: 90 centre point, 1 coincident, 1 point on line, 182 other
  measures "d61" diameter of A205
sketch "Sketch7" plane through (-21.2132, 21.2132, 20) normal (-0.7071068, -0.7071068, 0) x (-0.7071068, 0.7071068, 0)
  line L0 (-127.5, 20) -> (-60, 20) projected
  line L1 (-60, 0) -> (-127.5, 0) projected
  line L2 (-127.5, 0) -> (-127.5, 20) projected
  line L3 (67.5, 20) -> (67.5, 0) projected
  line L4 (0, 20) -> (67.5, 20) projected
  line L5 (67.5, 0) -> (0, 0) projected
  line L6 (0, 20) -> (-60, 20) projected
  line L7 (-60, 0) -> (0, 0) projected
  line L8 (67.497, 20) -> (67.497, 0) projected
  line L9 (-127.5, 20) -> (67.497, 20)
  line L10 (67.497, 20) -> (67.497, 0)
  line L11 (67.497, 0) -> (-127.5, 0)
  line L12 (-127.5, 0) -> (-127.5, 20)
  point P0 (-30, 20)
  constraints: 8 end point, 2 parallel, 1 horizontal, 1 perpendicular
extrude "Extrusion4" add sketch "Sketch7" along normal blind 30
extrude "Extrusion5" cut sketch "Sketch6" against normal up to surface (20 mm away) contours A203
sketch "Sketch8" plane through (-42.4264, 0, 20) normal (-0.7071068, -0.7071068, 0) x (0, 0, -1)
  line L0 (0, 127.5) -> (0, -67.5) projected
  line L1 (20, -67.5) -> (20, 127.5) projected
  line L2 (0, 30) -> (20, 30)
  line L3 (0, 20) -> (0, 40) projected
  line L4 (10, 30) -> (10, -37.5)
  line L5 (10, 30) -> (10, 97.5)
  line L6 (20, 45.1646) -> (0, 45.1646) projected
  line L7 (10, 30) -> (77.5, 30) construction
  circle A0 centre (10, -37.5) radius 3
  circle A1 centre (10, 30) radius 3
  circle A2 centre (10, 97.5) radius 3
  dimension "d72" = 67.5
  dimension "d73" = 67.5
  dimension "d74" = 90
  dimension "d75" = 6
  dimension "d76" = 6
  dimension "d77" = 6
  constraints: 8 end point, 3 centre point, 3 coincident, 3 perpendicular, 2 midpoint, 1 horizontal, 1 vertical
  measures "d72" distance of L4.start L4.end
  measures "d73" distance of L4.start L5.end
  measures "d74" angle of L7 L5
  measures "d75" diameter of A0
  measures "d76" diameter of A1
  measures "d77" diameter of A2
extrude "Extrusion7" cut sketch "Sketch8" against normal blind 30 contours A0 | A2
extrude "Extrusion8" cut sketch "Sketch8" against normal blind 10 contours A1 L2 L5 | L5 L2 A1 | L2 L4 A1 | L2 A1 L4
thread "Thread1" size "M6x1" class "6H" standard "ANSI Metric M Profile" full length
thread "Thread2" size "M6x1" class "6H" standard "ANSI Metric M Profile" full length
thread "Thread3" size "M6x1" class "6H" standard "ANSI Metric M Profile" full length
sketch "Sketch9" plane through (-14.1421, -14.1421, 10) normal (-0.7071068, -0.7071068, 0) x (-0.7071068, 0.7071068, 0)
  point P0 (0, 0)
hole "Hole1" at (-14.1421, -14.1421, 10) direction (0.7071068, 0.7071068, 0) diameter 4.917 depth 3 tip angle 120 thread size "M6x1" class "6H" standard "ISO Metric profile"
sketch "Sketch10" plane through (47.7297, -47.7297, 10) normal (-0.7071068, -0.7071068, 0) x (-0.7071068, 0.7071068, 0)
  point P0 (0, 0)
hole "Hole3" at (47.7297, -47.7297, 10) direction (0.7071068, 0.7071068, 0) diameter 4.917 depth 3 tip angle 120 thread size "M6x1" class "6H" standard "ISO Metric profile"
sketch "Sketch11" plane through (-47.7297, 47.7297, 10) normal (-0.7071068, -0.7071068, 0) x (-0.7071068, 0.7071068, 0)
  point P0 (0, 0)
hole "Hole5" at (-47.7297, 47.7297, 10) direction (0.7071068, 0.7071068, 0) diameter 4.917 depth 3 tip angle 120 thread size "M6x1" class "6H" standard "ISO Metric profile"
equation "\"d0\" = da_da"
equation "\"d1\" = da_b"
equation "\"d3\" = da_dw"
equation "\"da_da\" = 204"
equation "\"da_b\" = 20"
equation "\"da_dw\" = 200"
body "Solid1"
body "Srf1"
